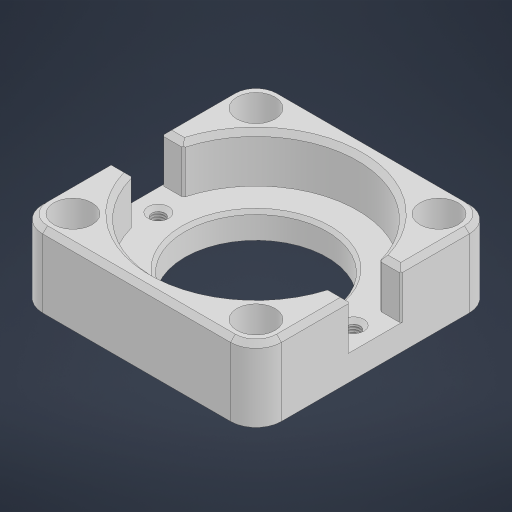
# Autodesk Inventor part: TH1-001
Saved by Autodesk Inventor 2024.3 (Build 283343000, 343)
## iProperties
Created: 2025-03-15
Part Number: TH1-001
Material: Generic
Document SubType Name: Modeling
Designer: fablabadmin
Density: 1 g/cm^3
Appearance: Default
Author: fablabadmin
Autodesk Inventor part; units mm, degrees
ref_plane "YZ Plane" through (0, 0, 0) normal (1, 0, 0) x (0, 1, 0)
ref_plane "XZ Plane" through (0, 0, 0) normal (0, 1, 0) x (-1, 0, 0)
ref_plane "XY Plane" through (0, 0, 0) normal (0, 0, 1) x (1, 0, 0)
sketch "Sketch1" plane through (0, 0, 0) normal (0, 1, 0) x (-1, 0, 0)
  line L0 (-37.5, 37.5) -> (37.5, 37.5)
  line L1 (37.5, 37.5) -> (37.5, -37.5)
  line L2 (37.5, -37.5) -> (-37.5, -37.5)
  line L3 (-37.5, -37.5) -> (-37.5, 37.5)
  line L4 (-37.5, 37.5) -> (37.5, -37.5) construction
  line L5 (37.5, 37.5) -> (-37.5, -37.5) construction
  line L6 (-28.75, 28.75) -> (28.75, 28.75) construction
  line L7 (28.75, 28.75) -> (28.75, -28.75) construction
  line L8 (28.75, -28.75) -> (-28.75, -28.75) construction
  line L9 (-28.75, -28.75) -> (-28.75, 28.75) construction
  line L10 (-28.75, 28.75) -> (28.75, -28.75) construction
  line L11 (28.75, 28.75) -> (-28.75, -28.75) construction
  circle A0 centre (0, 0) radius 22.325
  circle A1 centre (0, 0) radius 31.875
  line L12 (52.5, 0) -> (-52.5, 0) construction
  line L13 (0, -52.5) -> (0, 52.5) construction
  line L14 (-52.5, 0) -> (52.5, 0) construction
  line L15 (37.5, -8) -> (30.8548, -8)
  line L16 (37.5, 8) -> (30.8548, 8)
  line L17 (-37.5, -8) -> (-30.8548, -8)
  line L18 (-37.5, 8) -> (-30.8548, 8)
  point P0 (30.665, 0)
  point P1 (-30.665, 0)
  dimension "d2" = 63.75
  dimension "d0" = 75
  dimension "d1" = 44.65
  dimension "d3" = 57.5
  dimension "d4" = 61.33
  dimension "d7" = 16
  constraints: 34 end point, 9 symmetric about line, 6 coincident, 4 midpoint, 4 parallel, 4 point on line, 3 horizontal, 3 perpendicular, 1 centre point, 3 other
  measures "d0" distance of L2.end L0.start
  measures "d1" diameter of A0
  measures "d3" distance of L8.end L6.start
  measures "d4" distance of point (-30.665, 0) point (30.665, 0)
  measures "d7" distance between parallel lines of L16 L15
extrude "Extrusion1" add sketch "Sketch1" against normal blind 23
extrude "Extrusion2" cut sketch "Sketch1" against normal blind 15 contours L18 A1 L17 L3 | L1 L15 A1 L16 | A1
hole "Hole1" at (-28.75, 0, -28.75) at (28.75, 0, -28.75) at (28.75, 0, 28.75) at (-28.75, 0, 28.75) direction (0, -1, 0) diameter 6.5 end through all counterbore diameter 12 counterbore depth 12
sketch "Sketch2" plane through (0, -15, 0) normal (0, 1, 0) x (1, 0, 0)
  point P0 (0, 0)
  point P1 (-30.665, 0)
  point P2 (30.665, 0)
hole "Hole2" at (-30.665, -15, 0) at (30.665, -15, 0) direction (0, -1, 0) diameter 4.134 end through all countersink diameter 6.5 countersink angle 90 thread size "M5x0.8" class "6H" standard "ISO Metric profile"
fillet "Fillet1" radius 8 4 edges at (-37.5, -11.5, 37.5) (-37.5, -11.5, -37.5) (37.5, -11.5, -37.5) (37.5, -11.5, 37.5)
chamfer "Chamfer1" distance 1.5 angle 45 16 edges at (-37.5, 0, -18.75) (-35.1569, 0, -35.1569) (0, 0, -37.5) (35.1569, 0, -35.1569) (37.5, 0, -18.75) (0, 0, -31.875) (-34.1774, 0, -8) (34.1774, 0, -8) (34.1774, 0, 8) (37.5, 0, 18.75) (35.1569, 0, 35.1569) (0, 0, 37.5) (-35.1569, 0, 35.1569) (-37.5, 0, 18.75) (0, 0, 31.875) (-34.1774, 0, 8)
chamfer "Chamfer2" distance 1 angle 45 1 edges at (22.325, -15, 0)
chamfer "Chamfer3" distance 0.5 angle 45 14 edges at (-37.5, -8.25, -8) (-30.8548, -8.25, -8) (-30.8548, -8.25, 8) (-37.5, -8.25, 8) (30.8548, -8.25, -8) (37.5, -8.25, -8) (37.5, -8.25, 8) (30.8548, -8.25, 8) (28.75, -23, -32) (-28.75, -23, -32) (28.75, -23, 25.5) (-28.75, -23, 25.5) (30.665, -23, -2.067) (-30.665, -23, -2.067)
body "Solid1"
